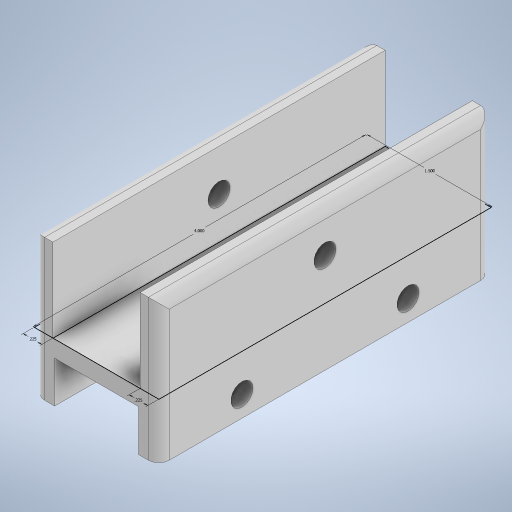
# Autodesk Inventor part: Rail Clip
Saved by Autodesk Inventor 2024.1 (Build 281209000, 209)
## iProperties
Created: 2022-02-14
Part Number: Rail Clip
Material: Generic
Document SubType Name: Modeling
Designer: Beaucage
Density: 1 g/cm^3
Appearance: Default
Author: Beaucage
Autodesk Inventor part; units mm, degrees
ref_plane "YZ Plane" through (0, 0, 0) normal (1, 0, 0) x (0, 1, 0)
ref_plane "XZ Plane" through (0, 0, 0) normal (0, 1, 0) x (-1, 0, 0)
ref_plane "XY Plane" through (0, 0, 0) normal (0, 0, 1) x (1, 0, 0)
sketch "Sketch1" plane through (0, 0, 0) normal (0, 1, 0) x (-1, 0, 0)
  line L0 (0, 0) -> (38.1, 0)
  line L1 (38.1, 0) -> (38.1, -101.6)
  line L2 (38.1, -101.6) -> (0, -101.6)
  line L3 (0, -101.6) -> (0, 0)
  line L4 (38.1, -101.6) -> (32.385, -101.6)
  line L5 (32.385, -101.6) -> (32.385, 0)
  line L6 (32.385, 0) -> (38.1, 0)
  line L7 (38.1, 0) -> (38.1, -101.6)
  line L8 (0, -101.6) -> (5.715, -101.6)
  line L9 (5.715, -101.6) -> (5.715, 0)
  line L10 (5.715, 0) -> (0, 0)
  line L11 (0, 0) -> (0, -101.6)
  dimension "d0" = 38.1
  dimension "d1" = 101.6
  dimension "d2" = 5.715
  dimension "d3" = 5.715
  constraints: 24 end point, 6 parallel, 3 horizontal, 3 perpendicular, 2 point on line
  measures "d0" distance of L1.end L2.end
  measures "d1" distance of L0.end L1.end
  measures "d2" distance of L5.end L6.end
  measures "d3" distance of L10.end L9.end
extrude "Extrusion1" add sketch "Sketch1" along normal blind 25.4 contours L0 L9 L2 L3 | L0 L1 L2 L5
extrude "Extrusion2" add sketch "Sketch1" against normal blind 5.08
sketch "Sketch2" plane through (0, 25.4, 0) normal (1, 0, 0) x (0, 0, -1)
  line L0 (101.6, 0) -> (0, 0) projected
  line L1 (50.8, 0) -> (50.8, -12.7)
  point P0 (0, -25.4)
  dimension "d8" = 12.7
  constraints: 2 end point, 1 midpoint, 1 vertical
  measures "d8" distance of L1.start L1.end
hole "Hole1" at (0, 12.7, -50.8) direction (-1, 0, 0) diameter 6.7564 end through all start extended yes clearance for "Socket Head Cap Screw" size "1/4" standard "Ansi Unified Screw Threads"
sketch "Sketch3" plane through (0, -5.08, 0) normal (0, -1, 0) x (1, 0, 0)
  line L0 (0, 0) -> (0, -101.6) projected
  line L1 (0, 0) -> (-6.223, 0)
  line L2 (-6.223, 0) -> (-6.223, -101.6)
  line L3 (-6.223, -101.6) -> (0, -101.6)
  line L4 (0, -101.6) -> (0, 0)
  line L5 (-38.1, -101.6) -> (-38.1, 0) projected
  line L6 (-38.1, 0) -> (-31.877, 0)
  line L7 (-31.877, 0) -> (-31.877, -101.6)
  line L8 (-31.877, -101.6) -> (-38.1, -101.6)
  line L9 (-38.1, -101.6) -> (-38.1, 0)
  dimension "d16" = 6.223
  dimension "d17" = 101.6
  dimension "d18" = 6.223
  constraints: 16 end point, 4 parallel, 2 horizontal, 2 perpendicular, 1 point on line
  measures "d16" distance of L3.end L2.end
  measures "d17" distance of L2.end L1.end
  measures "d18" distance of L7.end L8.end
extrude "Extrusion3" add sketch "Sketch3" along normal blind 12.7
sketch "Sketch4" plane through (-38.1, 25.4, -101.6) normal (-1, 0, 0) x (0, 0, 1)
  line L0 (101.6, -43.18) -> (101.6, 0) projected
  line L1 (101.6, -43.18) -> (76.2, -43.18)
  line L2 (76.2, -43.18) -> (76.2, -36.83)
  line L3 (76.2, -36.83) -> (101.6, -36.83)
  line L4 (101.6, -36.83) -> (101.6, -43.18)
  line L5 (0, -43.18) -> (0, 0) projected
  line L6 (0, -43.18) -> (25.4, -43.18)
  line L7 (25.4, -43.18) -> (25.4, -36.83)
  line L8 (25.4, -36.83) -> (0, -36.83)
  line L9 (0, -36.83) -> (0, -43.18)
  point P0 (101.6, -25.4)
  dimension "d21" = 25.4
  dimension "d22" = 6.35
  dimension "d23" = 25.4
  constraints: 16 end point, 4 parallel, 2 horizontal, 2 perpendicular, 1 point on line
  measures "d21" distance of L2.end L3.end
  measures "d22" distance of L1.end L2.end
  measures "d23" distance of L8.end L7.end
hole "Hole2" at (-38.1, -11.43, -25.4) at (-38.1, -11.43, -76.2) direction (1, 0, 0) diameter 6.7564 end through all clearance for "Socket Head Cap Screw" size "1/4" standard "Ansi Unified Screw Threads"
fillet "Fillet1" radius 3.175 6 edges at (-38.1, 3.81, 0) (-38.1, 25.4, -50.8) (0, 3.81, 0) (0, 25.4, -50.8) (0, 3.81, -101.6) (-38.1, 3.81, -101.6)
body "Solid1"
